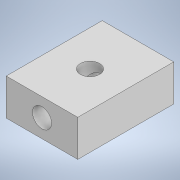
# Autodesk Inventor part: MM3_track
Saved by Autodesk Inventor 2021 (Build 250183000, 183)
## iProperties
Created: 2021-02-23
Part Number: MM3_track
Material: Generic
Document SubType Name: Modeling
Designer: dsdan
Density: 1 g/cm^3
Appearance: Default
Author: dsdan
Autodesk Inventor part; units mm, degrees
ref_plane "YZ Plane" through (0, 0, 0) normal (1, 0, 0) x (0, 1, 0)
ref_plane "XZ Plane" through (0, 0, 0) normal (0, 1, 0) x (-1, 0, 0)
ref_plane "XY Plane" through (0, 0, 0) normal (0, 0, 1) x (1, 0, 0)
sketch "Sketch1" plane through (0, 0, 0) normal (0, 1, 0) x (-1, 0, 0)
  line L0 (-7.45, 10) -> (-7.45, -10)
  line L1 (-7.45, -10) -> (7.45, -10)
  line L2 (7.45, -10) -> (7.45, 10)
  line L3 (7.45, 10) -> (-7.45, 10)
  line L4 (-7.45, 10) -> (7.45, -10) construction
  line L5 (-7.45, -10) -> (7.45, 10) construction
  point P0 (0, 0)
  dimension "d0" = 14.9
  dimension "d1" = 20
  constraints: 12 end point, 2 midpoint, 2 parallel, 1 perpendicular, 1 vertical
  measures "d0" distance of L1.end L0.end
  measures "d1" distance of L1.end L2.end
extrude "Extrusion1" add sketch "Sketch1" along normal blind 7.6
sketch "Sketch2" plane through (-7.45, 0, 10) normal (0, 0, 1) x (1, 0, 0)
  line L0 (14.9, 0) -> (0, 0) projected
  line L1 (14.9, 7.6) -> (0, 7.6) projected
  line L2 (0, 0) -> (14.9, 7.6) construction
  line L3 (0, 7.6) -> (14.9, 0) construction
  circle A0 centre (7.45, 3.8) radius 2
  point P0 (7.45, 0)
  dimension "d4" = 4
  constraints: 4 end point, 1 centre point, 1 midpoint
  measures "d4" diameter of A0
extrude "Extrusion2" cut sketch "Sketch2" against normal through all
sketch "Sketch3" plane through (0, 7.6, 0) normal (0, 1, 0) x (1, 0, 0)
  circle A0 centre (0, 0) radius 2
  dimension "d7" = 4
  constraints: 1 centre point, 1 coincident
  measures "d7" diameter of A0
extrude "Extrusion3" cut sketch "Sketch3" against normal through all
body "Solid1"
